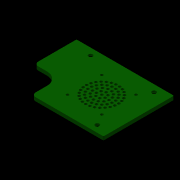
# Autodesk Inventor part: hw_DAA - PCB Lemo
Saved by Autodesk Inventor 2018 (Build 220112000, 112)
## iProperties
Created: 2024-03-13
Part Number: hw_DAA - PCB Lemo
Material: PCB
Document SubType Name: Modeling
Designer: cda1
Density: 4 g/cm^3
Appearance: PCB
Author: cda1
Autodesk Inventor part; units mm, degrees
ref_plane "YZ Plane" through (0, 0, 0) normal (1, 0, 0) x (0, 1, 0)
ref_plane "XZ Plane" through (0, 0, 0) normal (0, 1, 0) x (-1, 0, 0)
ref_plane "XY Plane" through (0, 0, 0) normal (0, 0, 1) x (1, 0, 0)
sketch "Boceto1" plane through (0, 0, 0) normal (0, 0, 1) x (1, 0, 0)
  line L0 (-26, 17) -> (26, 17)
  line L1 (26, 17) -> (26, -17)
  line L2 (26, -17) -> (-26, -17)
  line L3 (-26, -17) -> (-26, 17)
  line L4 (-26, 17) -> (26, -17) construction
  line L5 (26, 17) -> (-26, -17) construction
  point P0 (0, 0)
  dimension "d0" = 52
  dimension "d1" = 34
  constraints: 12 end point, 2 midpoint, 2 parallel, 1 horizontal, 1 perpendicular
  measures "d0" distance of L1.end L2.end
  measures "d1" distance of L0.end L1.end
extrude "Extrusión1" add sketch "Boceto1" against normal blind 1.742
fillet "Empalme1" radius 0.5 4 edges at (26, 17, -0.871) (-26, 17, -0.871) (-26, -17, -0.871) (26, -17, -0.871)
sketch "Boceto2" plane through (0, 0, -1.742) normal (0, 0, -1) x (-1, 0, 0)
  circle A0 centre (19.65, -11) radius 4
  point P0 (0, 0)
  dimension "d5" = 8
  constraints: 1 centre point, 1 coincident
  measures "d5" diameter of A0
extrude "Extrusión2" cut sketch "Boceto2" against normal through all
sketch "Boceto3" plane through (0, 0, 0) normal (0, 0, 1) x (1, 0, 0)
  line L0 (26, -16.5) -> (26, 16.5) projected
  line L1 (26, 17) -> (22.748, 17)
  line L2 (22.748, 17) -> (22.748, -17)
  line L3 (22.748, -17) -> (26, -17)
  line L4 (26, -17) -> (26, 17)
  line L5 (25.5, -17) -> (-25.5, -17) projected
  point P0 (0, 0)
  point P1 (25.5, 17)
  dimension "d8" = 3.252
  constraints: 8 end point, 3 point on line, 2 parallel, 1 horizontal, 1 perpendicular
  measures "d8" distance of L3.end L2.end
extrude "Extrusión3" cut sketch "Boceto3" against normal through all
sketch "Boceto4" plane through (0, 0, -1.742) normal (0, 0, -1) x (-1, 0, 0)
  circle A0 centre (18, -9.5) radius 4 construction
  arc A1 (18, -3.5) -> (12, -9.5) centre (18, -9.5) ccw
  line L0 (12, -9.5) -> (12, -17)
  line L1 (18, -3.5) -> (26, -3.5)
  line L2 (26, -16.5) -> (26, 16.5) projected
  arc A2 (25.5, -17) -> (26, -16.5) centre (25.5, -16.5) ccw projected
  line L3 (-25.5, -17) -> (25.5, -17) projected
  line L4 (25.5, -17) -> (12, -17)
  line L5 (26, -16.5) -> (26, -3.5)
  point P0 (0, 0)
  dimension "d13" = 12
  dimension "d63" = 8
  dimension "d64" = 7.5
  constraints: 8 end point, 2 centre point, 2 point on circle, 2 tangent, 1 coincident, 1 collinear, 1 horizontal, 1 perpendicular, 1 point on line, 1 vertical
  measures "d13" diameter of A1
  measures "d63" distance from line of L2 A0.centre
  measures "d64" distance from line of L3 A0.centre
extrude "Extrusión4" cut sketch "Boceto4" against normal through all
fillet "Empalme2" radius 2 2 edges at (-12, -17, -0.871) (-26, -3.5, -0.871)
sketch "Boceto13" plane through (0, 0, -1.742) normal (0, 0, -1) x (-1, 0, 0)
  line L0 (-22.748, 17) -> (-22.748, -17) projected
  line L1 (-22.748, -17) -> (10, -17) projected
  line L2 (25.5, 17) -> (-22.748, 17) projected
  point P0 (0, 0)
  point P1 (-16.448, 13.678)
  point P2 (-16.448, -13.678)
  point P3 (14.152, 13.678)
  dimension "d52" = 6.3
  dimension "d53" = 3.322
  dimension "d54" = 3.322
  dimension "d62" = 30.6
  constraints: 1 horizontal alignment, 1 vertical alignment
  measures "d52" distance from line of L0 point (-16.448, -13.678)
  measures "d53" distance from line of L1 point (-16.448, -13.678)
  measures "d54" distance from line of L2 point (-16.448, 13.678)
  measures "d62" distance of point (-16.448, 13.678) point (14.152, 13.678)
hole "Agujero4" at (16.448, 13.678, -1.742) at (16.448, -13.678, -1.742) at (-14.152, 13.678, -1.742) direction (0, 0, 1) diameter 2 end through all countersink diameter 4 countersink angle 90
fillet "Empalme4" radius 0.5 2 edges at (22.748, 17, -0.871) (22.748, -17, -0.871)
sketch "Boceto15" plane through (0, 0, -1.742) normal (0, 0, -1) x (-1, 0, 0)
  line L0 (25.994, -1.5) -> (25.994, 16.5)
  line L1 (26, -1.5) -> (26, 16.5) projected
  arc A0 (23.994, -3.5) -> (25.994, -1.5) centre (23.994, -1.5) ccw
  line L2 (18, -3.5) -> (24, -3.5) projected
  arc A1 (24, -3.5) -> (26, -1.5) centre (24, -1.5) ccw projected
  arc A2 (25.994, 16.5) -> (25.494, 17) centre (25.494, 16.5) ccw
  line L3 (25.5, 17) -> (-22.248, 17) projected
  arc A3 (26, 16.5) -> (25.5, 17) centre (25.5, 16.5) ccw projected
  line L4 (23.994, -3.5) -> (24, -3.5)
  arc A4 (23.997, -3.5) -> (26, -1.5) centre (24, -1.5) ccw
  arc A5 (25.994, 16.4228) -> (25.497, 17) centre (25.5, 16.5) ccw
  line L5 (26, 16.5) -> (26, -1.5)
  line L6 (25.497, 17) -> (25.5, 17)
  point P0 (0, 0)
  dimension "d68" = 0.006
  dimension "d69" = 4
  dimension "d70" = 1
  dimension "d71" = 4
  dimension "d72" = 1
  constraints: 12 point on circle, 8 end point, 8 tangent, 5 point on line, 4 centre point, 2 collinear, 1 vertical
  measures "d68" distance between parallel lines of L0 L1
  measures "d69" diameter of A0
  measures "d70" diameter of A2
  measures "d71" diameter of A4
  measures "d72" diameter of A5
extrude "Extrusión8" cut sketch "Boceto15" against normal up to surface (1.742 mm away)
sketch "Boceto16" plane through (0, 0, -1.742) normal (0, 0, -1) x (-1, 0, 0)
  arc A0 (22.252, -3.5) -> (24.252, -1.5) centre (22.252, -1.5) ccw
  arc A1 (24.252, 16.5) -> (23.752, 17) centre (23.752, 16.5) ccw
  line L0 (24.252, -1.5) -> (24.252, 16.5)
  line L1 (18, -3.5) -> (23.997, -3.5) projected
  line L2 (25.497, 17) -> (-22.248, 17) projected
  arc A2 (25.994, 16.5) -> (25.497, 17) centre (25.494, 16.5) ccw projected
  arc A3 (24, -3.5) -> (25.994, -1.5) centre (23.994, -1.5) ccw projected
  line L3 (23.994, -3.5) -> (22.252, -3.5)
  line L4 (23.752, 17) -> (25.497, 17)
  arc A4 (23.994, -3.5) -> (25.994, -1.5) centre (23.994, -1.5) ccw
  arc A5 (25.994, 16.5) -> (25.494, 17) centre (25.494, 16.5) ccw
  line L5 (25.994, -1.5) -> (25.994, 16.5)
  point P0 (0, 0)
  dimension "d75" = 4
  dimension "d76" = 1
  dimension "d78" = 1.742
  constraints: 10 point on circle, 8 end point, 6 tangent, 4 centre point, 4 point on line, 2 coincident, 2 vertical, 1 collinear, 1 concentric
  measures "d75" diameter of A0
  measures "d76" diameter of A1
  measures "d78" distance between parallel lines of L5 L0
extrude "Extrusión9" cut sketch "Boceto16" against normal up to surface (1.742 mm away)
sketch "Boceto17" plane through (0, 0, -1.742) normal (0, 0, -1) x (-1, 0, 0)
  point P0 (0, 0)
  point P1 (-13.203, 8.255)
  point P2 (3.307, 8.255)
  point P3 (-4.948, 0)
  point P4 (-13.203, -8.255)
  point P5 (3.307, -8.255)
  point P6 (-12.58, -1.346)
  point P7 (-12.685, 0.451)
  point P8 (-12.372, 2.223)
  point P9 (-11.66, 3.875)
  point P10 (-10.585, 5.318)
  point P11 (-9.207, 6.475)
  point P12 (-7.599, 7.283)
  point P13 (-5.848, 7.698)
  point P14 (-4.048, 7.698)
  point P15 (-2.297, 7.283)
  point P16 (-0.689, 6.475)
  point P17 (0.689, 5.318)
  point P18 (1.764, 3.875)
  point P19 (2.476, 2.223)
  point P20 (2.789, 0.451)
  point P21 (2.684, -1.346)
  point P22 (2.168, -3.07)
  point P23 (1.268, -4.628)
  point P24 (0.034, -5.937)
  point P25 (-1.47, -6.926)
  point P26 (-3.161, -7.541)
  point P27 (-4.948, -7.75)
  point P28 (-6.735, -7.541)
  point P29 (-8.426, -6.926)
  point P30 (-9.93, -5.937)
  point P31 (-11.164, -4.628)
  point P32 (-12.064, -3.07)
  point P33 (-9.102, 4.154)
  point P34 (-7.615, 5.235)
  point P35 (-5.867, 5.803)
  point P36 (-4.029, 5.803)
  point P37 (-2.281, 5.235)
  point P38 (-0.794, 4.154)
  point P39 (0.287, 2.667)
  point P40 (0.855, 0.919)
  point P41 (0.855, -0.919)
  point P42 (0.287, -2.667)
  point P43 (-0.794, -4.154)
  point P44 (-2.281, -5.235)
  point P45 (-4.029, -5.803)
  point P46 (-5.867, -5.803)
  point P47 (-7.615, -5.235)
  point P48 (-9.102, -4.154)
  point P49 (-10.183, -2.667)
  point P50 (-10.751, -0.919)
  point P51 (-10.751, 0.919)
  point P52 (-10.183, 2.667)
  point P53 (-8.688, 1.418)
  point P54 (-7.6, 2.994)
  point P55 (-5.905, 3.884)
  point P56 (-3.991, 3.884)
  point P57 (-2.296, 2.994)
  point P58 (-1.208, 1.418)
  point P59 (-0.977, -0.482)
  point P60 (-1.656, -2.272)
  point P61 (-3.089, -3.542)
  point P62 (-4.948, -4)
  point P63 (-6.807, -3.542)
  point P64 (-8.24, -2.272)
  point P65 (-8.919, -0.482)
  point P66 (-6.609, 1.325)
  point P67 (-4.948, 2.125)
  point P68 (-3.287, 1.325)
  point P69 (-2.876, -0.473)
  point P70 (-4.026, -1.915)
  point P71 (-5.87, -1.915)
  point P72 (-7.02, -0.473)
hole "Agujero5" at (13.203, 8.255, -1.742) at (-3.307, 8.255, -1.742) at (4.948, 0, -1.742) at (13.203, -8.255, -1.742) at (-3.307, -8.255, -1.742) at (12.58, -1.346, -1.742) at (12.685, 0.451, -1.742) at (12.372, 2.223, -1.742) at (11.66, 3.875, -1.742) at (10.585, 5.318, -1.742) at (9.207, 6.475, -1.742) at (7.599, 7.283, -1.742) at (5.848, 7.698, -1.742) at (4.048, 7.698, -1.742) at (2.297, 7.283, -1.742) at (0.689, 6.475, -1.742) at (-0.689, 5.318, -1.742) at (-1.764, 3.875, -1.742) at (-2.476, 2.223, -1.742) at (-2.789, 0.451, -1.742) at (-2.684, -1.346, -1.742) at (-2.168, -3.07, -1.742) at (-1.268, -4.628, -1.742) at (-0.034, -5.937, -1.742) at (1.47, -6.926, -1.742) at (3.161, -7.541, -1.742) at (4.948, -7.75, -1.742) at (6.735, -7.541, -1.742) at (8.426, -6.926, -1.742) at (9.93, -5.937, -1.742) at (11.164, -4.628, -1.742) at (12.064, -3.07, -1.742) at (9.102, 4.154, -1.742) at (7.615, 5.235, -1.742) at (5.867, 5.803, -1.742) at (4.029, 5.803, -1.742) at (2.281, 5.235, -1.742) at (0.794, 4.154, -1.742) at (-0.287, 2.667, -1.742) at (-0.855, 0.919, -1.742) at (-0.855, -0.919, -1.742) at (-0.287, -2.667, -1.742) at (0.794, -4.154, -1.742) at (2.281, -5.235, -1.742) at (4.029, -5.803, -1.742) at (5.867, -5.803, -1.742) at (7.615, -5.235, -1.742) at (9.102, -4.154, -1.742) at (10.183, -2.667, -1.742) at (10.751, -0.919, -1.742) direction (0, 0, 1) diameter 1.3 end through all and at (10.751, 0.919, -1.742) (10.183, 2.667, -1.742) (8.688, 1.418, -1.742) (7.6, 2.994, -1.742) (5.905, 3.884, -1.742) (3.991, 3.884, -1.742) (2.296, 2.994, -1.742) (1.208, 1.418, -1.742) (0.977, -0.482, -1.742) (1.656, -2.272, -1.742) (3.089, -3.542, -1.742) (4.948, -4, -1.742) (6.807, -3.542, -1.742) (8.24, -2.272, -1.742) (8.919, -0.482, -1.742) (6.609, 1.325, -1.742) (4.948, 2.125, -1.742) (3.287, 1.325, -1.742) (2.876, -0.473, -1.742) (4.026, -1.915, -1.742) (5.87, -1.915, -1.742) (7.02, -0.473, -1.742)
